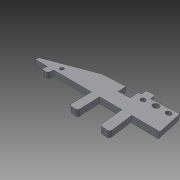
# Autodesk Inventor part: x_motor_upper_nut_stop
Saved by Autodesk Inventor 2014 (Build 180170000, 170)
## iProperties
Created: 2013-12-01
Part Number: x_motor_upper_nut_stop
Material: Generic
Document SubType Name: Modeling
Designer: buben
Density: 1 g/cm^3
Appearance: Anodized - Dark Gray
Author: buben
Subject: Laser Cutted
Autodesk Inventor part; units mm, degrees
ref_plane "YZ Plane" through (0, 0, 0) normal (1, 0, 0) x (0, 1, 0)
ref_plane "XZ Plane" through (0, 0, 0) normal (0, 1, 0) x (-1, 0, 0)
ref_plane "XY Plane" through (0, 0, 0) normal (0, 0, 1) x (1, 0, 0)
sketch "Sketch1" plane through (0, 0, 0) normal (0, 0, 1) x (1, 0, 0)
  line L0 (0, 4) -> (0, 0)
  line L1 (0, 0) -> (125, 0)
  line L2 (125, 0) -> (125, 23)
  line L3 (57, 23) -> (0, 4)
  line L4 (81, 23) -> (81, 14)
  line L5 (81, 14) -> (92, 14)
  line L6 (92, 14) -> (92, 23)
  line L7 (125, 23) -> (92, 23)
  line L8 (81, 23) -> (57, 23)
  circle A0 centre (99.5, 18.5) radius 2.25
  circle A1 centre (119.5, 18.5) radius 2.25
  circle A2 centre (28.2, 6) radius 2.25
  circle A3 centre (28.2, 6) radius 4.5 construction
  point P0 (92, 18.5)
  dimension "d0" = 4
  dimension "d1" = 125
  dimension "d2" = 9
  dimension "d3" = 11
  dimension "d4" = 33
  dimension "d5" = 24
  dimension "d6" = 23
  dimension "d7" = 4.5
  dimension "d8" = 4.5
  dimension "d9" = 5.5
  dimension "d10" = 20
  dimension "d11" = 4.5
  dimension "d12" = 9
  dimension "d13" = 6
  dimension "d14" = 28.2
  constraints: 18 end point, 6 perpendicular, 4 centre point, 3 parallel, 2 horizontal alignment, 1 coincident, 1 collinear, 1 midpoint, 1 vertical
  measures "d0" distance of L0.start L0.end
  measures "d1" distance of L0.end L1.end
  measures "d2" distance of L5.end L6.end
  measures "d3" distance of L4.end L5.end
  measures "d4" distance of L2.end L6.end
  measures "d5" distance of L4.start L3.start
  measures "d6" distance of L1.end L2.end
  measures "d7" diameter of A1
  measures "d8" diameter of A0
  measures "d9" distance from line of L2 A1.centre
  measures "d10" distance of A1.centre A0.centre
  measures "d11" diameter of A2
  measures "d12" diameter of A3
  measures "d13" distance from line of L1 A2.centre
  measures "d14" distance from line of L0 A2.centre
extrude "Extrusion1" add sketch "Sketch1" along normal blind 6
sketch "Sketch2" plane through (0, 0, 6) normal (0, 0, 1) x (1, 0, 0)
  line L0 (0, 0) -> (125, 0) projected
  line L1 (125, 0) -> (125, 23) projected
  line L2 (125, 23) -> (92, 23) projected
  line L3 (17, 0) -> (25, 0)
  line L4 (25, 0) -> (25, -4)
  line L5 (23, -6) -> (19, -6)
  line L6 (17, -4) -> (17, 0)
  line L7 (96, 0) -> (104, 0)
  line L8 (104, 0) -> (104, -19)
  line L9 (102, -21) -> (98, -21)
  line L10 (96, -19) -> (96, 0)
  line L11 (68, 0) -> (76, 0)
  line L12 (76, 0) -> (76, -19)
  line L13 (74, -21) -> (70, -21)
  line L14 (68, -19) -> (68, 0)
  line L15 (94.5, 23) -> (102.5, 23)
  line L16 (102.5, 23) -> (102.5, 27)
  line L17 (100.5, 29) -> (96.5, 29)
  line L18 (94.5, 27) -> (94.5, 23)
  arc A0 (17, -4) -> (19, -6) centre (19, -4) ccw
  arc A1 (23, -6) -> (25, -4) centre (23, -4) ccw
  arc A2 (96, -19) -> (98, -21) centre (98, -19) ccw
  arc A3 (102, -21) -> (104, -19) centre (102, -19) ccw
  arc A4 (68, -19) -> (70, -21) centre (70, -19) ccw
  arc A5 (74, -21) -> (76, -19) centre (74, -19) ccw
  arc A6 (96.5, 29) -> (94.5, 27) centre (96.5, 27) ccw
  arc A7 (102.5, 27) -> (100.5, 29) centre (100.5, 27) ccw
  dimension "d17" = 2
  dimension "d18" = 17
  dimension "d20" = 8
  dimension "d21" = 8
  dimension "d22" = 8
  dimension "d24" = 6
  dimension "d25" = 43
  dimension "d26" = 20
  dimension "d29" = 8
  dimension "d32" = 22.5
  dimension "d40" = 6
  dimension "d41" = 2
  dimension "d42" = 2
  dimension "d45" = 21
  constraints: 32 end point, 16 point on circle, 16 tangent, 8 centre point, 8 parallel, 5 equal radius, 4 horizontal, 4 perpendicular, 4 point on line, 1 collinear
  measures "d17" radius of A0
  measures "d18" distance from line of L6 L0.start
  measures "d20" distance between parallel lines of L4 L6
  measures "d21" distance between parallel lines of L12 L14
  measures "d22" distance between parallel lines of L8 L10
  measures "d24" distance between parallel lines of L0 L5
  measures "d25" distance between parallel lines of L14 L4
  measures "d26" distance between parallel lines of L10 L12
  measures "d29" distance between parallel lines of L16 L18
  measures "d32" distance between parallel lines of L1 L16
  measures "d40" distance between parallel lines of L15 L17
  measures "d41" radius of A7
  measures "d42" radius of A6
  measures "d45" distance between parallel lines of L0 L13
sketch "Sketch3" plane through (0, 0, 6) normal (0, 0, 1) x (1, 0, 0)
  circle A0 centre (119.5, 18.5) radius 2.25 projected
  circle A1 centre (109.5, 19.099) radius 2.75
  circle A2 centre (86.5, 19.099) radius 7.5 construction
  dimension "d35" = 5.5
  dimension "d36" = 15
  dimension "d37" = 10
  constraints: 2 centre point, 1 horizontal alignment
  measures "d35" diameter of A1
  measures "d36" diameter of A2
  measures "d37" horizontal distance of A0.centre A1.centre
extrude "Extrusion3" cut sketch "Sketch3" against normal blind 6 contours A1
extrude "Extrusion4" add sketch "Sketch2" against normal blind 6
body "Solid1"
